Autodesk Fusion 360 part; units mm, degrees
note: some values were not read from the file. Chosen so that the rebuilt part matches the saved one: which bodies a step acts on.
(part 3 of 3)
  line L675 (-34.1437, -40.1697) -> (-31.5928, -38.6629) construction
  line L676 (-31.5928, -38.6629) -> (-29.8835, -37.7222) construction
  spline S219 degree 3 poles (-29.8835, -37.7222) (-29.2848, -37.3926) (-28.7626, -37.0952) (-27.9251, -36.6064) knots 0 0 0 0 1 1 1 1
  line L677 (-29.8835, -37.7222) -> (-29.2848, -37.3926) construction
  line L678 (-29.2848, -37.3926) -> (-28.7626, -37.0952) construction
  line L679 (-28.7626, -37.0952) -> (-27.9251, -36.6064) construction
  spline S220 degree 3 poles (-27.9251, -36.6064) (-26.9048, -36.0111) (-26.2975, -35.6653) (-26.2208, -35.636) knots 0 0 0 0 1 1 1 1
  line L680 (-27.9251, -36.6064) -> (-26.9048, -36.0111) construction
  line L681 (-26.9048, -36.0111) -> (-26.2975, -35.6653) construction
  line L682 (-26.2975, -35.6653) -> (-26.2208, -35.636) construction
  spline S221 degree 3 poles (-26.2208, -35.636) (-26.2038, -35.6296) (-26.0008, -35.7304) (-25.6667, -35.9114) knots 0 0 0 0 1 1 1 1
  line L683 (-26.2208, -35.636) -> (-26.2038, -35.6296) construction
  line L684 (-26.2038, -35.6296) -> (-26.0008, -35.7304) construction
  line L685 (-26.0008, -35.7304) -> (-25.6667, -35.9114) construction
  spline S222 degree 3 poles (-25.7428, -37.5545) (-24.4673, -38.1995) (-21.2005, -40.009) (-19.166, -41.1975) knots 0 0 0 0 1 1 1 1
  line L686 (-25.7428, -37.5545) -> (-24.4673, -38.1995) construction
  line L687 (-24.4673, -38.1995) -> (-21.2005, -40.009) construction
  line L688 (-21.2005, -40.009) -> (-19.166, -41.1975) construction
  spline S223 degree 3 poles (-19.166, -41.1975) (-18.513, -41.5789) (-18.0684, -41.8524) (-18.0809, -41.8648) knots 0 0 0 0 1 1 1 1
  line L689 (-19.166, -41.1975) -> (-18.513, -41.5789) construction
  line L690 (-18.513, -41.5789) -> (-18.0684, -41.8524) construction
  line L691 (-18.0684, -41.8524) -> (-18.0809, -41.8648) construction
  spline S224 degree 3 poles (-18.0809, -41.8648) (-18.1008, -41.8847) (-18.5997, -41.6495) (-19.6279, -41.1354) knots 0 0 0 0 1 1 1 1
  line L692 (-18.0809, -41.8648) -> (-18.1008, -41.8847) construction
  line L693 (-18.1008, -41.8847) -> (-18.5997, -41.6495) construction
  line L694 (-18.5997, -41.6495) -> (-19.6279, -41.1354) construction
  spline S225 degree 3 poles (-19.6279, -41.1354) (-20.9362, -40.4812) (-21.7257, -40.0612) (-22.0995, -39.8204) knots 0 0 0 0 1 1 1 1
  line L695 (-19.6279, -41.1354) -> (-20.9362, -40.4812) construction
  line L696 (-20.9362, -40.4812) -> (-21.7257, -40.0612) construction
  line L697 (-21.7257, -40.0612) -> (-22.0995, -39.8204) construction
  spline S226 degree 3 poles (-22.0995, -39.8204) (-22.4079, -39.6216) (-22.6658, -39.4794) (-23.2646, -39.1777) knots 0 0 0 0 1 1 1 1
  line L698 (-22.0995, -39.8204) -> (-22.4079, -39.6216) construction
  line L699 (-22.4079, -39.6216) -> (-22.6658, -39.4794) construction
  line L700 (-22.6658, -39.4794) -> (-23.2646, -39.1777) construction
  spline S227 degree 3 poles (-23.2646, -39.1777) (-24.0824, -38.7657) (-24.7899, -38.3231) (-25.4378, -38.0628) knots 0 0 0 0 1 1 1 1
  line L701 (-23.2646, -39.1777) -> (-24.0824, -38.7657) construction
  line L702 (-24.0824, -38.7657) -> (-24.7899, -38.3231) construction
  line L703 (-24.7899, -38.3231) -> (-25.4378, -38.0628) construction
  spline S228 degree 3 poles (-25.4378, -38.0628) (-25.9181, -37.8698) (-25.5452, -37.9991) (-26.072, -37.7234) knots 0 0 0 0 1 1 1 1
  line L704 (-25.4378, -38.0628) -> (-25.9181, -37.8698) construction
  line L705 (-25.9181, -37.8698) -> (-25.5452, -37.9991) construction
  line L706 (-25.5452, -37.9991) -> (-26.072, -37.7234) construction
  spline S229 degree 3 poles (-26.072, -37.7234) (-26.2446, -37.6817) (-26.575, -37.8504) (-26.6249, -37.87) knots 0 0 0 0 1 1 1 1
  line L707 (-26.072, -37.7234) -> (-26.2446, -37.6817) construction
  line L708 (-26.2446, -37.6817) -> (-26.575, -37.8504) construction
  line L709 (-26.575, -37.8504) -> (-26.6249, -37.87) construction
  spline S230 degree 3 poles (-26.6249, -37.87) (-26.7469, -37.9178) (-27.123, -38.1964) (-28.1297, -38.7533) knots 0 0 0 0 1 1 1 1
  line L710 (-26.6249, -37.87) -> (-26.7469, -37.9178) construction
  line L711 (-26.7469, -37.9178) -> (-27.123, -38.1964) construction
  line L712 (-27.123, -38.1964) -> (-28.1297, -38.7533) construction
  spline S231 degree 3 poles (-28.1297, -38.7533) (-31.2174, -40.4614) (-33.3065, -41.7393) (-33.8578, -41.9941) knots 0 0 0 0 1 1 1 1
  line L713 (-28.1297, -38.7533) -> (-31.2174, -40.4614) construction
  line L714 (-31.2174, -40.4614) -> (-33.3065, -41.7393) construction
  line L715 (-33.3065, -41.7393) -> (-33.8578, -41.9941) construction
  spline S232 degree 3 poles (-33.8578, -41.9941) (-34.2176, -42.1604) (-34.3437, -42.1895) (-34.3635, -42.1108) knots 0 0 0 0 1 1 1 1
  line L716 (-33.8578, -41.9941) -> (-34.2176, -42.1604) construction
  line L717 (-34.2176, -42.1604) -> (-34.3437, -42.1895) construction
  line L718 (-34.3437, -42.1895) -> (-34.3635, -42.1108) construction
  spline S233 degree 3 poles (-34.3635, -42.1108) (-34.3767, -42.058) (-34.3713, -42.0507) (-34.2413, -41.9471) knots 0 0 0 0 1 1 1 1
  line L719 (-34.3635, -42.1108) -> (-34.3767, -42.058) construction
  line L720 (-34.3767, -42.058) -> (-34.3713, -42.0507) construction
  line L721 (-34.3713, -42.0507) -> (-34.2413, -41.9471) construction
  spline S234 degree 3 poles (-34.2413, -41.9471) (-33.9434, -41.7095) (-33.4673, -41.4178) (-32.2551, -40.7301) knots 0 0 0 0 1 1 1 1
  line L722 (-34.2413, -41.9471) -> (-33.9434, -41.7095) construction
  line L723 (-33.9434, -41.7095) -> (-33.4673, -41.4178) construction
  line L724 (-33.4673, -41.4178) -> (-32.2551, -40.7301) construction
  spline S235 degree 3 poles (-32.2551, -40.7301) (-31.7688, -40.4542) (-30.8392, -39.9239) (-30.1893, -39.5516) knots 0 0 0 0 1 1 1 1
  line L725 (-32.2551, -40.7301) -> (-31.7688, -40.4542) construction
  line L726 (-31.7688, -40.4542) -> (-30.8392, -39.9239) construction
  line L727 (-30.8392, -39.9239) -> (-30.1893, -39.5516) construction
  spline S236 degree 3 poles (-30.1893, -39.5516) (-27.8491, -38.2112) (-27.325, -37.9184) (-26.658, -37.5787) knots 0 0 0 0 1 1 1 1
  line L728 (-30.1893, -39.5516) -> (-27.8491, -38.2112) construction
  line L729 (-27.8491, -38.2112) -> (-27.325, -37.9184) construction
  line L730 (-27.325, -37.9184) -> (-26.658, -37.5787) construction
  spline S237 degree 3 poles (-26.658, -37.5787) (-26.4, -37.4473) (-26.2063, -37.3585) (-26.178, -37.3585) knots 0 0 0 0 1 1 1 1
  line L731 (-26.658, -37.5787) -> (-26.4, -37.4473) construction
  line L732 (-26.4, -37.4473) -> (-26.2063, -37.3585) construction
  line L733 (-26.2063, -37.3585) -> (-26.178, -37.3585) construction
  spline S238 degree 3 poles (-26.178, -37.3585) (-26.15, -37.3585) (-25.9704, -37.4394) (-25.7428, -37.5545) knots 0 0 0 0 1 1 1 1
  line L734 (-26.178, -37.3585) -> (-26.15, -37.3585) construction
  line L735 (-26.15, -37.3585) -> (-25.9704, -37.4394) construction
  line L736 (-25.9704, -37.4394) -> (-25.7428, -37.5545) construction
  spline S239 degree 3 poles (-26.1154, -34.9158) (-25.8921, -34.9929) (-25.0226, -35.4205) (-24.4215, -35.7486) knots 0 0 0 0 1 1 1 1
  line L737 (-26.1154, -34.9158) -> (-25.8921, -34.9929) construction
  line L738 (-25.8921, -34.9929) -> (-25.0226, -35.4205) construction
  line L739 (-25.0226, -35.4205) -> (-24.4215, -35.7486) construction
  spline S240 degree 3 poles (-24.4215, -35.7486) (-24.1169, -35.9149) (-19.3681, -38.5832) (-18.571, -39.0359) knots 0 0 0 0 1 1 1 1
  line L740 (-24.4215, -35.7486) -> (-24.1169, -35.9149) construction
  line L741 (-24.1169, -35.9149) -> (-19.3681, -38.5832) construction
  line L742 (-19.3681, -38.5832) -> (-18.571, -39.0359) construction
  spline S241 degree 3 poles (-18.571, -39.0359) (-17.405, -39.6982) (-16.5172, -40.2351) (-16.5439, -40.2618) knots 0 0 0 0 1 1 1 1
  line L743 (-18.571, -39.0359) -> (-17.405, -39.6982) construction
  line L744 (-17.405, -39.6982) -> (-16.5172, -40.2351) construction
  line L745 (-16.5172, -40.2351) -> (-16.5439, -40.2618) construction
  spline S242 degree 3 poles (-16.5439, -40.2618) (-16.5585, -40.2764) (-16.8618, -40.1363) (-17.3563, -39.8865) knots 0 0 0 0 1 1 1 1
  line L746 (-16.5439, -40.2618) -> (-16.5585, -40.2764) construction
  line L747 (-16.5585, -40.2764) -> (-16.8618, -40.1363) construction
  line L748 (-16.8618, -40.1363) -> (-17.3563, -39.8865) construction
  spline S243 degree 3 poles (-17.3563, -39.8865) (-18.1679, -39.4765) (-19.8684, -38.5676) (-24.1622, -36.2488) knots 0 0 0 0 1 1 1 1
  line L749 (-17.3563, -39.8865) -> (-18.1679, -39.4765) construction
  line L750 (-18.1679, -39.4765) -> (-19.8684, -38.5676) construction
  line L751 (-19.8684, -38.5676) -> (-24.1622, -36.2488) construction
  line L752 (-24.1622, -36.2488) -> (-25.9936, -35.2597)
  line L753 (-25.9936, -35.2597) -> (-26.7073, -35.6419)
  spline S244 degree 3 poles (-26.7073, -35.6419) (-27.8903, -36.2753) (-29.1019, -36.9382) (-31.7923, -38.4243) knots 0 0 0 0 1 1 1 1
  line L754 (-26.7073, -35.6419) -> (-27.8903, -36.2753) construction
  line L755 (-27.8903, -36.2753) -> (-29.1019, -36.9382) construction
  line L756 (-29.1019, -36.9382) -> (-31.7923, -38.4243) construction
  spline S245 degree 3 poles (-31.7923, -38.4243) (-33.9077, -39.5928) (-34.4259, -39.8735) (-34.9611, -40.1412) knots 0 0 0 0 1 1 1 1
  line L757 (-31.7923, -38.4243) -> (-33.9077, -39.5928) construction
  line L758 (-33.9077, -39.5928) -> (-34.4259, -39.8735) construction
  line L759 (-34.4259, -39.8735) -> (-34.9611, -40.1412) construction
  spline S246 degree 3 poles (-34.9611, -40.1412) (-35.4286, -40.375) (-35.6579, -40.4604) (-35.7384, -40.4306) knots 0 0 0 0 1 1 1 1
  line L760 (-34.9611, -40.1412) -> (-35.4286, -40.375) construction
  line L761 (-35.4286, -40.375) -> (-35.6579, -40.4604) construction
  line L762 (-35.6579, -40.4604) -> (-35.7384, -40.4306) construction
  spline S247 degree 3 poles (-35.7384, -40.4306) (-35.8101, -40.4041) (-35.7817, -40.3579) (-35.6306, -40.2549) knots 0 0 0 0 1 1 1 1
  line L763 (-35.7384, -40.4306) -> (-35.8101, -40.4041) construction
  line L764 (-35.8101, -40.4041) -> (-35.7817, -40.3579) construction
  line L765 (-35.7817, -40.3579) -> (-35.6306, -40.2549) construction
  spline S248 degree 3 poles (-35.6306, -40.2549) (-34.7769, -39.6734) (-28.9995, -36.3439) (-26.879, -35.2113) knots 0 0 0 0 1 1 1 1
  line L766 (-35.6306, -40.2549) -> (-34.7769, -39.6734) construction
  line L767 (-34.7769, -39.6734) -> (-28.9995, -36.3439) construction
  line L768 (-28.9995, -36.3439) -> (-26.879, -35.2113) construction
  spline S249 degree 3 poles (-26.879, -35.2113) (-26.2698, -34.8859) (-26.2377, -34.8735) (-26.1154, -34.9158) knots 0 0 0 0 1 1 1 1
  line L769 (-26.879, -35.2113) -> (-26.2698, -34.8859) construction
  line L770 (-26.2698, -34.8859) -> (-26.2377, -34.8735) construction
  line L771 (-26.2377, -34.8735) -> (-26.1154, -34.9158) construction
  spline S250 degree 3 poles (-25.9832, -34.1748) (-25.3061, -34.5036) (-23.6316, -35.4014) (-22.711, -35.9292) knots 0 0 0 0 1 1 1 1
  line L772 (-25.9832, -34.1748) -> (-25.3061, -34.5036) construction
  line L773 (-25.3061, -34.5036) -> (-23.6316, -35.4014) construction
  line L774 (-23.6316, -35.4014) -> (-22.711, -35.9292) construction
  spline S251 degree 3 poles (-22.711, -35.9292) (-22.1528, -36.2492) (-21.7622, -36.4638) (-20.8765, -36.9368) knots 0 0 0 0 1 1 1 1
  line L775 (-22.711, -35.9292) -> (-22.1528, -36.2492) construction
  line L776 (-22.1528, -36.2492) -> (-21.7622, -36.4638) construction
  line L777 (-21.7622, -36.4638) -> (-20.8765, -36.9368) construction
  spline S252 degree 3 poles (-20.8765, -36.9368) (-18.5007, -38.2058) (-16.0738, -39.5933) (-16.1307, -39.6502) knots 0 0 0 0 1 1 1 1
  line L778 (-20.8765, -36.9368) -> (-18.5007, -38.2058) construction
  line L779 (-18.5007, -38.2058) -> (-16.0738, -39.5933) construction
  line L780 (-16.0738, -39.5933) -> (-16.1307, -39.6502) construction
  spline S253 degree 3 poles (-16.1307, -39.6502) (-16.1794, -39.699) (-17.4464, -39.0334) (-21.7111, -36.7188) knots 0 0 0 0 1 1 1 1
  line L781 (-16.1307, -39.6502) -> (-16.1794, -39.699) construction
  line L782 (-16.1794, -39.699) -> (-17.4464, -39.0334) construction
  line L783 (-17.4464, -39.0334) -> (-21.7111, -36.7188) construction
  spline S254 degree 3 poles (-21.7111, -36.7188) (-23.0163, -36.0104) (-23.7493, -35.6248) (-25.0769, -34.9479) knots 0 0 0 0 1 1 1 1
  line L784 (-21.7111, -36.7188) -> (-23.0163, -36.0104) construction
  line L785 (-23.0163, -36.0104) -> (-23.7493, -35.6248) construction
  line L786 (-23.7493, -35.6248) -> (-25.0769, -34.9479) construction
  spline S255 degree 3 poles (-25.0769, -34.9479) (-25.5965, -34.6831) (-26.0305, -34.4663) (-26.0413, -34.4663) knots 0 0 0 0 1 1 1 1
  line L787 (-25.0769, -34.9479) -> (-25.5965, -34.6831) construction
  line L788 (-25.5965, -34.6831) -> (-26.0305, -34.4663) construction
  line L789 (-26.0305, -34.4663) -> (-26.0413, -34.4663) construction
  spline S256 degree 3 poles (-26.0413, -34.4663) (-26.0521, -34.4663) (-26.7797, -34.8596) (-27.6582, -35.3402) knots 0 0 0 0 1 1 1 1
  line L790 (-26.0413, -34.4663) -> (-26.0521, -34.4663) construction
  line L791 (-26.0521, -34.4663) -> (-26.7797, -34.8596) construction
  line L792 (-26.7797, -34.8596) -> (-27.6582, -35.3402) construction
  spline S257 degree 3 poles (-27.6582, -35.3402) (-30.8435, -37.0829) (-31.2781, -37.3146) (-32.1025, -37.7095) knots 0 0 0 0 1 1 1 1
  line L793 (-27.6582, -35.3402) -> (-30.8435, -37.0829) construction
  line L794 (-30.8435, -37.0829) -> (-31.2781, -37.3146) construction
  line L795 (-31.2781, -37.3146) -> (-32.1025, -37.7095) construction
  spline S258 degree 3 poles (-32.1025, -37.7095) (-32.1596, -37.7368) (-32.3046, -37.8236) (-32.4248, -37.9024) knots 0 0 0 0 1 1 1 1
  line L796 (-32.1025, -37.7095) -> (-32.1596, -37.7368) construction
  line L797 (-32.1596, -37.7368) -> (-32.3046, -37.8236) construction
  line L798 (-32.3046, -37.8236) -> (-32.4248, -37.9024) construction
  spline S259 degree 3 poles (-32.4248, -37.9024) (-32.8253, -38.165) (-33.2586, -38.4152) (-34.23, -38.9449) knots 0 0 0 0 1 1 1 1
  line L799 (-32.4248, -37.9024) -> (-32.8253, -38.165) construction
  line L800 (-32.8253, -38.165) -> (-33.2586, -38.4152) construction
  line L801 (-33.2586, -38.4152) -> (-34.23, -38.9449) construction
  spline S260 degree 3 poles (-34.23, -38.9449) (-34.9008, -39.3107) (-35.3686, -39.5733) (-35.6981, -39.769) knots 0 0 0 0 1 1 1 1
  line L802 (-34.23, -38.9449) -> (-34.9008, -39.3107) construction
  line L803 (-34.9008, -39.3107) -> (-35.3686, -39.5733) construction
  line L804 (-35.3686, -39.5733) -> (-35.6981, -39.769) construction
  spline S261 degree 3 poles (-35.6981, -39.769) (-35.9605, -39.9249) (-36.109, -39.9572) (-36.1564, -39.8685) knots 0 0 0 0 1 1 1 1
  line L805 (-35.6981, -39.769) -> (-35.9605, -39.9249) construction
  line L806 (-35.9605, -39.9249) -> (-36.109, -39.9572) construction
  line L807 (-36.109, -39.9572) -> (-36.1564, -39.8685) construction
  spline S262 degree 3 poles (-36.1564, -39.8685) (-36.1729, -39.8378) (-36.1639, -39.8232) (-36.0784, -39.7403) knots 0 0 0 0 1 1 1 1
  line L808 (-36.1564, -39.8685) -> (-36.1729, -39.8378) construction
  line L809 (-36.1729, -39.8378) -> (-36.1639, -39.8232) construction
  line L810 (-36.1639, -39.8232) -> (-36.0784, -39.7403) construction
  spline S263 degree 3 poles (-36.0784, -39.7403) (-35.8332, -39.5028) (-35.075, -39.0535) (-31.6684, -37.1272) knots 0 0 0 0 1 1 1 1
  line L811 (-36.0784, -39.7403) -> (-35.8332, -39.5028) construction
  line L812 (-35.8332, -39.5028) -> (-35.075, -39.0535) construction
  line L813 (-35.075, -39.0535) -> (-31.6684, -37.1272) construction
  spline S264 degree 3 poles (-31.6684, -37.1272) (-29.645, -35.9831) (-29.0122, -35.6236) (-27.9003, -34.987) knots 0 0 0 0 1 1 1 1
  line L814 (-31.6684, -37.1272) -> (-29.645, -35.9831) construction
  line L815 (-29.645, -35.9831) -> (-29.0122, -35.6236) construction
  line L816 (-29.0122, -35.6236) -> (-27.9003, -34.987) construction
  spline S265 degree 3 poles (-27.9003, -34.987) (-26.7253, -34.3142) (-26.2796, -34.0695) (-26.2302, -34.0701) knots 0 0 0 0 1 1 1 1
  line L817 (-27.9003, -34.987) -> (-26.7253, -34.3142) construction
  line L818 (-26.7253, -34.3142) -> (-26.2796, -34.0695) construction
  line L819 (-26.2796, -34.0695) -> (-26.2302, -34.0701) construction
  spline S266 degree 3 poles (-26.2302, -34.0701) (-26.2125, -34.0704) (-26.1014, -34.1175) (-25.9832, -34.1748) knots 0 0 0 0 1 1 1 1
  line L820 (-26.2302, -34.0701) -> (-26.2125, -34.0704) construction
  line L821 (-26.2125, -34.0704) -> (-26.1014, -34.1175) construction
  line L822 (-26.1014, -34.1175) -> (-25.9832, -34.1748) construction
  line L823 (-46, -28) -> (-6, -28)
  line L824 (-6, -28) -> (-6, -30)
  line L825 (-46, -30) -> (-46, -28)
  line L826 (-46, -57) -> (-46, -55)
  line L827 (-6, -55) -> (-6, -57)
  line L828 (-6, -57) -> (-46, -57)
  line L829 (-46, -18) -> (-46, -16)
  line L830 (-46, -16) -> (-6, -16)
  line L831 (-6, -16) -> (-6, -18)
  line L832 (-6, -18) -> (-46, -18)
  line L833 (-46, -22) -> (-46, -20)
  line L834 (-46, -20) -> (-6, -20)
  line L835 (-6, -20) -> (-6, -22)
  line L836 (-6, -22) -> (-46, -22)
  line L837 (-46, -59) -> (-6, -59)
  line L838 (-6, -59) -> (-6, -61)
  line L839 (-6, -61) -> (-46, -61)
  line L840 (-46, -61) -> (-46, -59)
  line L841 (-46, -26) -> (-46, -24)
  line L842 (-46, -24) -> (-6, -24)
  line L843 (-6, -24) -> (-6, -26)
  line L844 (-6, -26) -> (-46, -26)
  line L845 (-46, -63) -> (-6, -63)
  line L846 (-6, -63) -> (-6, -65)
  line L847 (-6, -65) -> (-46, -65)
  line L848 (-46, -65) -> (-46, -63)
fillet "Raccordo2" radius 1 1 edges at (0, 35, 24) on bodies 1
fillet "Raccordo2" radius 1 1 edges at (52, 35, 24) on bodies 1
fillet "Raccordo2" radius 1 1 edges at (0, 35, 0) on bodies 1
fillet "Raccordo2" radius 1 1 edges at (52, 35, 0) on bodies 1
chamfer "Smusso1" distance 5 angle 10 1 edges at (26, 9.8, 22.5) measured on face at (18, 3.2667, 22.5) on bodies 1
chamfer "Smusso1" distance 5 angle 10 1 edges at (26, 9.8, 1.5) measured on face at (34, 3.2667, 1.5) on bodies 1
extrude "Estrusione1''" add sketch "Schizzo12" along normal blind 1.5 separate body contours S0 S1 S2 S3 S4 S5 S6 S7 S8 S9 S10 S11 S12 S13 S14 S15 S16 L57 | S17 S18 S19 S20 S21 S22 S23 S24 S25 S26 S27 | S28 S29 S30 S31 S32 S33 L109 L110 S34 S35 S36 S37 S38 S39 | S40 S41 S42 S43 S44 S45 S46 S47 S48 S49 S50 S51 | S52 S53 S54 S55 S56 S57 S58 S59 S60 S61 S62 S63 S64 S65 | S66 S67 S68 S69 L219 L220 S70 S71 S72 S73 S74 S75 | S76 S77 S78 S79 S80 S81 S82 S83 S84 S85 S86 | S87 S88 L278 L279 S89 S90 S91 S92 S93 S94 S95 S96 S97 | S98 S99 S100 S101 L319 L320 S102 S103 S104 S105 S106 S107 S108 | S109 S110 S111 L351 L352 S112 S113 S114 S115 S116 S117 S118 S119 S120 | S121 S122 S123 S124 S125 S126 S127 S128 S129 | S130 S131 S132 S133 S134 S135 S136 S137 S138 S139 | S140 S141 S142 S143 L449 L450 S144 S145 S146 S147 S148 | S149 S150 S151 S152 S153 S154 S155 S156 S157 S158 S159 | S160 S161 S162 S163 S164 S165 S166 S167 | S168 S169 S170 S171 S172 S173 S174 | S175 S176 S177 S178 | S179 S180 S181 S182 S183 S184 S185 S186 S187 S188 S189 S190 S191 S192 L598 | S193 S194 S195 S196 S197 S198 S199 S200 S201 S202 S203 S204 S205 S206 | S207 S208 S209 S210 S211 S212 S213 S214 S215 S216 S217 S218 S219 S220 S221 | S222 S223 S224 S225 S226 S227 S228 S229 S230 S231 S232 S233 S234 S235 S236 S237 S238 | S239 S240 S241 S242 S243 L752 L753 S244 S245 S246 S247 S248 S249 | S250 S251 S252 S253 S254 S255 S256 S257 S258 S259 S260 S261 S262 S263 S264 S265 S266 makes body 8 at (25.9318, 50.5832, 24.6667) makes body 9 at (28.2629, 48.3854, 24.6667) makes body 10 at (27.7751, 44.7717, 24.6667) makes body 11 at (27.951, 41.5705, 24.6667) makes body 12 at (19.8854, 40.7808, 24.6667) makes body 13 at (20.3981, 37.4305, 24.6667) makes body 14 at (33.9207, 41.2115, 24.6667) makes body 15 at (31.4377, 43.1547, 24.6667) makes body 16 at (26.6178, 43.376, 24.6667) makes body 17 at (28.7885, 47.8461, 24.6667) makes body 18 at (27.1529, 50.2145, 24.6667) makes body 19 at (26.2858, 51.3984, 24.6667) makes body 20 at (25.6562, 48.2288, 24.6667) makes body 21 at (29.9249, 46.8858, 24.6667) makes body 22 at (25.1361, 41.9533, 24.6667) makes body 23 at (25.0536, 38.7124, 24.6667) makes body 24 at (27.7095, 35.6634, 24.6667) makes body 25 at (24.808, 36.3798, 24.6667) makes body 26 at (30.1939, 41.669, 24.6667) makes body 27 at (27.7664, 43.114, 24.6667) makes body 28 at (27.3189, 46.6764, 24.6667) makes body 29 at (25.1472, 49.3364, 25.1667) makes body 30 at (26.0319, 52.1935, 24.6667) in component "Componente_Logo"
ref_plane "Piano di lavoro3" through (26, 70, 12) normal (0, 1, 0) x (-1, 0, 0)
sketch "Schizzo13" plane through (26, 70, 12) normal (0, 1, 0) x (1, 0, 0)
  line L0 (26, -12) -> (-26, -12)
  line L1 (-26, -12) -> (-26, 12)
  line L2 (-26, 12) -> (26, 12)
  line L3 (26, 12) -> (26, -12)
  dimension "d99" = 24
  dimension "d100" = 52
  constraint horizontal L0
  constraint perpendicular L0 L1
  constraint perpendicular L1 L2
  constraint perpendicular L0 L3
  measures "d99" distance of L0.start L2.end
  measures "d100" distance of L0.start L0.end
extrude "Estrusione9" add sketch "Schizzo13" along normal blind 2 separate body makes body 31
sketch "Schizzo14" plane through (0, 72, 0) normal (0, 1, 0) x (-1, 0, 0)
  line L0 (-52, 0) -> (0, 0)
  line L1 (0, 0) -> (0, 24)
  line L2 (0, 24) -> (-52, 24)
  line L3 (-52, 24) -> (-52, 0)
  circle A0 centre (-50, 12.7) radius 0.65
  circle A1 centre (-2, 12.7) radius 0.65
  circle A2 centre (-2, 12.7) radius 0.65
  dimension "d122" = 2
  constraint equal A0 A1
  constraint equal A1 A2
  constraint coincident A1.centre A2.centre
  constraint horizontal A0.centre A1.centre
  measures "d122" distance of L3 A0.centre
hole "Foratura2" at (50, 72, 12.7) at (2, 72, 12.7) direction (0, -1, 0) diameter 1.3 depth 2.097 tip angle 180 countersink diameter 1.6 countersink angle 90 bodies 31
sketch "Schizzo15" plane through (0, 70, 0) normal (0, -1, 0) x (1, 0, 0)
  circle A0 centre (50, 12.7) radius 0.65
  circle A1 centre (2, 12.7) radius 0.65
  line L0 (0, 0) -> (52, 0)
  line L1 (52, 0) -> (52, 24)
  line L2 (52, 24) -> (0, 24)
  line L3 (0, 24) -> (0, 0)
  line L4 (5, 9.85) -> (47, 9.85)
  line L5 (47, 9.85) -> (47, 7.85)
  line L6 (47, 7.85) -> (5, 7.85)
  line L7 (5, 7.85) -> (5, 9.85)
  line L8 (5, 9.85) -> (47, 9.85)
  line L9 (5, 7.85) -> (5, 9.85)
  constraint horizontal L4
  constraint vertical L5
  constraint horizontal L6
  constraint vertical L7
  constraint equal L4 L8
  constraint equal L7 L9
  constraint coincident L4.start L7.end
extrude "Estrusione10" add sketch "Schizzo15" along normal blind 1.4 contours L4 L5 L6 L7 L8 L9 bodies 31
fillet "Raccordo3" radius 1 1 edges at (52, 71, 24) on bodies 31
fillet "Raccordo3" radius 1 1 edges at (0, 71, 24) on bodies 31
fillet "Raccordo3" radius 1 1 edges at (52, 71, 0) on bodies 31
fillet "Raccordo3" radius 1 1 edges at (0, 71, 0) on bodies 31
copy_body "Corpo->Comp1" bodies 31 removing the originals makes body 32 in component "Coperchio"
copy_body "Corpo->Comp2" bodies 1 removing the originals makes body 33 in component "Case"
other "Lavorazione mesh di base1"
other "Corpo->Comp1'"
other "Modifica1" in component "pcb-MultiRom"
other "Lavorazione mesh di base2"
other "Corpo->Comp2'"
other "Modifica1'" in component "edgeconnector-Model"
other "Modifica2" in component "edgeconnector-Model"
combine "Combina2" operation add target body 33 tool bodies 4 7 5 6 2 3 in component "Case"
sketch "Schizzo16" plane through (0, 0, 24) normal (0, 0, 1) x (-1, 0, 0)
  line L0 (-16.0196, -48.0156) -> (-16.0196, -48.6944)
  line L1 (-17.5571, -48.6944) -> (-17.5571, -46.2033)
  spline S0 degree 2 poles (-17.5571, -46.2033) (-16.8532, -45.9324) (-16.0939, -45.9324) knots 0 0 0 1 1 1
  spline S1 degree 2 poles (-16.0939, -45.9324) (-15.19, -45.9324) (-14.6849, -46.6156) knots 0 0 0 1 1 1
  spline S2 degree 2 poles (-14.6849, -46.6156) (-14.1799, -47.2988) (-14.1799, -48.4965) knots 0 0 0 1 1 1
  spline S3 degree 2 poles (-14.1799, -48.4965) (-14.1799, -49.6843) (-14.7346, -50.3675) knots 0 0 0 1 1 1
  spline S4 degree 2 poles (-14.7346, -50.3675) (-15.2893, -51.0507) (-16.2629, -51.0507) knots 0 0 0 1 1 1
  spline S5 degree 2 poles (-16.2629, -51.0507) (-16.9168, -51.0507) (-17.4809, -50.7257) knots 0 0 0 1 1 1
  line L2 (-17.4809, -50.7257) -> (-17.2047, -50.0935)
  spline S6 degree 2 poles (-17.2047, -50.0935) (-16.669, -50.3719) (-16.2445, -50.3719) knots 0 0 0 1 1 1
  spline S7 degree 2 poles (-16.2445, -50.3719) (-15.647, -50.3719) (-15.3092, -49.8807) knots 0 0 0 1 1 1
  spline S8 degree 2 poles (-15.3092, -49.8807) (-14.9715, -49.3894) (-14.9715, -48.4915) knots 0 0 0 1 1 1
  spline S9 degree 2 poles (-14.9715, -48.4915) (-14.9715, -46.6112) (-16.2022, -46.6112) knots 0 0 0 1 1 1
  spline S10 degree 2 poles (-16.2022, -46.6112) (-16.5151, -46.6112) (-16.802, -46.6906) knots 0 0 0 1 1 1
  line L3 (-16.802, -46.6906) -> (-16.802, -48.0156)
  line L4 (-16.802, -48.0156) -> (-16.0196, -48.0156)
  line L5 (-13.1262, -46.5373) -> (-13.1262, -46)
  line L6 (-13.1262, -46) -> (-10.4187, -46)
  line L7 (-10.4187, -46) -> (-10.4187, -46.5376)
  line L8 (-10.4187, -46.5376) -> (-11.3966, -46.6039)
  line L9 (-11.3966, -46.6039) -> (-11.3966, -50.3747)
  line L10 (-11.3966, -50.3747) -> (-10.4187, -50.441)
  line L11 (-10.4187, -50.441) -> (-10.4187, -50.9797)
  line L12 (-10.4187, -50.9797) -> (-13.1262, -50.9797)
  line L13 (-13.1262, -50.9797) -> (-13.1262, -50.4413)
  line L14 (-13.1262, -50.4413) -> (-12.1517, -50.3751)
  line L15 (-12.1517, -50.3751) -> (-12.1517, -46.6036)
  line L16 (-12.1517, -46.6036) -> (-13.1262, -46.5373)
  line L17 (-35.9453, -47.9983) -> (-35.2961, -47.9983)
  line L18 (-35.2961, -47.9983) -> (-35.2961, -46)
  line L19 (-35.2961, -46) -> (-34.5409, -46)
  line L20 (-34.5409, -46) -> (-34.5409, -50.9797)
  line L21 (-34.5409, -50.9797) -> (-35.792, -50.9797)
  spline S11 degree 2 poles (-35.792, -50.9797) (-37.5869, -50.9797) (-37.5869, -49.5355) knots 0 0 0 1 1 1
  spline S12 degree 2 poles (-37.5869, -49.5355) (-37.5869, -48.5363) (-36.6274, -48.1996) knots 0 0 0 1 1 1
  line L22 (-36.6274, -48.1996) -> (-37.9461, -46)
  line L23 (-37.9461, -46) -> (-37.1091, -46)
  line L24 (-37.1091, -46) -> (-35.9453, -47.9983)
  spline S13 degree 2 poles (-45.3576, -49.0077) (-45.3576, -49.2263) (-45.3766, -49.6687) knots 0 0 0 0.640385 0.640385 0.640385
  line L25 (-45.3766, -49.6687) -> (-44.5647, -46)
  line L26 (-44.5647, -46) -> (-43.9423, -46)
  line L27 (-43.9423, -46) -> (-43.1615, -49.596)
  spline S14 degree 2 poles (-43.1615, -49.596) (-43.1806, -49.2202) (-43.1806, -48.9646) knots 0.433911 0.433911 0.433911 1 1 1
  line L28 (-43.1806, -48.9646) -> (-43.1806, -46)
  line L29 (-43.1806, -46) -> (-42.5382, -46)
  line L30 (-42.5382, -46) -> (-42.5382, -50.9797)
  line L31 (-42.5382, -50.9797) -> (-43.4818, -50.9797)
  line L32 (-43.4818, -50.9797) -> (-44.2572, -47.2526)
  line L33 (-44.2572, -47.2526) -> (-45.0388, -50.9797)
  line L34 (-45.0388, -50.9797) -> (-46, -50.9797)
  line L35 (-46, -50.9797) -> (-46, -46)
  line L36 (-46, -46) -> (-45.3576, -46)
  line L37 (-45.3576, -46) -> (-45.3576, -49.0077)
  line L38 (-6, -30) -> (-46, -30)
  line L39 (-46, -55) -> (-6, -55)
  line L40 (-51, 0) -> (-51, -70)
  line L41 (-51, -70) -> (-1, -70)
  line L42 (-1, -70) -> (-1, 0)
  line L43 (-1, 0) -> (-51, 0)
  spline S15 degree 2 poles (-8.5566, -48.6203) (-9.4618, -48.3879) (-9.4618, -47.4715) knots 0.093077 0.093077 0.093077 1 1 1
  spline S16 degree 2 poles (-9.4618, -47.4715) (-9.4618, -46.7868) (-9.0172, -46.3934) knots 0 0 0 1 1 1
  spline S17 degree 2 poles (-9.0172, -46.3934) (-8.5725, -46) (-7.8154, -46) knots 0 0 0 1 1 1
  line L44 (-7.8154, -46) -> (-6, -46)
  line L45 (-6, -46) -> (-6, -50.9797)
  line L46 (-6, -50.9797) -> (-7.5273, -50.9797)
  spline S18 degree 2 poles (-7.5273, -50.9797) (-8.4582, -50.9797) (-8.8924, -50.6722) knots 0 0 0 1 1 1
  spline S19 degree 2 poles (-8.8924, -50.6722) (-9.3266, -50.3647) (-9.3266, -49.685) knots 0 0 0 1 1 1
  spline S20 degree 2 poles (-9.3266, -49.685) (-9.3266, -49.2344) (-9.0486, -48.9336) knots 0 0 0 1 1 1
  spline S21 degree 2 poles (-9.0486, -48.9336) (-8.8398, -48.7075) (-8.5566, -48.6203) knots 0 0 0 0.751565 0.751565 0.751565
  spline S22 degree 2 poles (-41.5117, -46.606) (-41.0372, -45.9324) (-40.1538, -45.9324) knots 0 0 0 1 1 1
  spline S23 degree 2 poles (-40.1538, -45.9324) (-38.3215, -45.9324) (-38.3215, -48.5032) knots 0 0 0 1 1 1
  spline S24 degree 2 poles (-38.3215, -48.5032) (-38.3215, -51.0575) (-40.1604, -51.0575) knots 0 0 0 1 1 1
  spline S25 degree 2 poles (-40.1604, -51.0575) (-41.0466, -51.0575) (-41.5164, -50.385) knots 0 0 0 1 1 1
  spline S26 degree 2 poles (-41.5164, -50.385) (-41.9861, -49.7124) (-41.9861, -48.4966) knots 0 0 0 1 1 1
  spline S27 degree 2 poles (-41.9861, -48.4966) (-41.9861, -47.2795) (-41.5117, -46.606) knots 0 0 0 1 1 1
  line L47 (-17.5571, -55) -> (-17.5571, -30) construction
  line L48 (-34.5409, -55) -> (-34.5409, -30) construction
  line L49 (-26, -52.5) -> (-14.5333, -38.625)
  line L50 (-26, -55) -> (-26, -30) construction
  line L51 (-14.5333, -38.625) -> (-26, -32.5)
  line L52 (-26, -52.5) -> (-37.4667, -38.625)
  line L53 (-37.4667, -38.625) -> (-26, -32.5)
  line L54 (-17.5571, -55) -> (-34.5409, -55) construction
  line L55 (-34.5409, -55) -> (-34.5409, -52.5) construction
  line L56 (-34.5409, -52.5) -> (-17.5571, -52.5) construction
  line L57 (-17.5571, -52.5) -> (-17.5571, -55) construction
  line L58 (-17.5571, -30) -> (-34.5409, -30) construction
  line L59 (-34.5409, -30) -> (-34.5409, -32.5) construction
  line L60 (-34.5409, -32.5) -> (-17.5571, -32.5) construction
  line L61 (-17.5571, -32.5) -> (-17.5571, -30) construction
  line L62 (-46, -28) -> (-6, -28)
  line L63 (-6, -28) -> (-6, -30)
  line L64 (-46, -30) -> (-46, -28)
  line L65 (-46, -57) -> (-46, -55)
  line L66 (-6, -55) -> (-6, -57)
  line L67 (-6, -57) -> (-46, -57)
  line L68 (-46, -18) -> (-46, -16)
  line L69 (-46, -16) -> (-6, -16)
  line L70 (-6, -16) -> (-6, -18)
  line L71 (-6, -18) -> (-46, -18)
  line L72 (-46, -22) -> (-46, -20)
  line L73 (-46, -20) -> (-6, -20)
  line L74 (-6, -20) -> (-6, -22)
  line L75 (-6, -22) -> (-46, -22)
  line L76 (-46, -59) -> (-6, -59)
  line L77 (-6, -59) -> (-6, -61)
  line L78 (-6, -61) -> (-46, -61)
  line L79 (-46, -61) -> (-46, -59)
  line L80 (-46, -26) -> (-46, -24)
  line L81 (-46, -24) -> (-6, -24)
  line L82 (-6, -24) -> (-6, -26)
  line L83 (-6, -26) -> (-46, -26)
  line L84 (-46, -63) -> (-6, -63)
  line L85 (-6, -63) -> (-6, -65)
  line L86 (-6, -65) -> (-46, -65)
  line L87 (-46, -65) -> (-46, -63)
  dimension "d129" = 18
  dimension "d139" = 18
  dimension "d140" = 13
  dimension "d141" = 13
  dimension "d142" = 2.5
  constraint coincident L39 L47.start
  constraint perpendicular L39 L47
  constraint coincident L39 L48.start
  constraint coincident L38 L48.end
  constraint perpendicular L38 L48
  constraint midpoint L39 L50.start
  constraint midpoint L38 L50.end
  constraint coincident L50 L51.end
  constraint coincident L49.start L50
  constraint collinear L1 L47
  constraint collinear L20 L48
  constraint horizontal L54
  constraint vertical L55
  constraint horizontal L56
  constraint vertical L57
  constraint coincident L48 L55.end
  constraint horizontal L58
  constraint vertical L59
  constraint horizontal L60
  constraint vertical L61
  constraint coincident L48 L59.end
  constraint coincident L51.end L60
  constraint coincident L49.start L56
  constraint equal L55 L59
  constraint collinear L38 L58
  measures "d129" distance of L49.start L52.end
  measures "d139" distance of L49.start L49.end
  measures "d140" distance of L51.end L49.end
  measures "d141" distance of L51.end L52.end
  measures "d142" distance of L47.end L60.end
extrude "Estrusione1'''" add sketch "Schizzo16" along normal blind 1.5 contours L49 L51 L52 L53 bodies 33 in component "Case"
sketch "Schizzo17" plane through (0, 0, 25.5) normal (0, 0, 1) x (-1, 0, 0)
  line L0 (-26, -52.5) -> (-14.5333, -38.625)
  line L1 (-14.5333, -38.625) -> (-26, -32.5)
  line L2 (-26, -32.5) -> (-37.4667, -38.625)
  line L3 (-37.4667, -38.625) -> (-26, -52.5)
  line L4 (-26, -52.5) -> (-26, -32.5) construction
  line L5 (-22.1778, -47.875) -> (-26, -45.8333)
  line L6 (-26, -45.8333) -> (-29.8222, -47.875)
  line L7 (-23.4519, -49.4167) -> (-26, -48.0556)
  line L8 (-26, -48.0556) -> (-28.5481, -49.4167)
  line L9 (-24.7259, -50.9583) -> (-26, -50.2778)
  line L10 (-26, -50.2778) -> (-27.2741, -50.9583)
  line L11 (-20.9037, -46.3333) -> (-26, -43.6111)
  line L12 (-31.0963, -46.3333) -> (-26, -43.6111)
  line L13 (-19.6296, -44.7917) -> (-26, -41.3889)
  line L14 (-26, -41.3889) -> (-32.3704, -44.7917)
  line L15 (-18.3556, -43.25) -> (-26, -39.1667)
  line L16 (-26, -39.1667) -> (-33.6444, -43.25)
  line L17 (-17.0815, -41.7083) -> (-26, -36.9444)
  line L18 (-26, -36.9444) -> (-34.9185, -41.7083)
  line L19 (-15.8074, -40.1667) -> (-26, -34.7222)
  line L20 (-26, -34.7222) -> (-36.1926, -40.1667)
  line L21 (-15.8074, -40.1667) -> (-17.0815, -41.7083)
  line L22 (-18.3556, -43.25) -> (-19.6296, -44.7917)
  line L23 (-20.9037, -46.3333) -> (-22.1778, -47.875)
  line L24 (-23.4519, -49.4167) -> (-24.7259, -50.9583)
  line L25 (-27.2741, -50.9583) -> (-28.5481, -49.4167)
  line L26 (-29.8222, -47.875) -> (-31.0963, -46.3333)
  line L27 (-32.3704, -44.7917) -> (-33.6444, -43.25)
  line L28 (-34.9185, -41.7083) -> (-36.1926, -40.1667)
  dimension "d132" = 2
  dimension "d133" = 2
  dimension "d134" = 2
  dimension "d135" = 2
  dimension "d136" = 2
  dimension "d137" = 2
  dimension "d138" = 2
  dimension "d143" = 2
  constraint coincident L0.start L3.end
  constraint coincident L1.end L2.start
  constraint coincident L0 L5.start
  constraint coincident L4 L5.end
  constraint coincident L3 L6.end
  constraint coincident L4 L7.end
  constraint coincident L0 L9.start
  constraint coincident L3 L10.end
  constraint parallel L1 L5
  constraint parallel L2 L6
  constraint parallel L5 L7
  constraint parallel L7 L9
  constraint coincident L4 L9.end
  constraint coincident L0 L7.start
  constraint equal L7 L8
  constraint coincident L0 L11.start
  constraint coincident L4 L11.end
  constraint coincident L3 L12.start
  constraint coincident L0 L13.start
  constraint coincident L4 L13.end
  constraint parallel L11 L13
  constraint coincident L3 L14.end
  constraint parallel L12 L14
  constraint parallel L5 L11
  constraint parallel L6 L12
  constraint coincident L0 L15.start
  constraint coincident L4 L15.end
  constraint parallel L13 L15
  constraint coincident L3 L16.end
  constraint coincident L0 L17.start
  constraint coincident L4 L17.end
  constraint parallel L15 L17
  constraint coincident L3 L18.end
  constraint parallel L14 L16
  constraint parallel L16 L18
  constraint coincident L0 L19.start
  constraint coincident L4 L19.end
  constraint coincident L3 L20.end
  constraint parallel L17 L19
  constraint parallel L18 L20
  constraint parallel L3 L25
  constraint equal L9 L10
  measures "d132" distance of L0.start L9.start
  measures "d133" distance of L5.start L7.start
  measures "d134" distance of L7.start L9.start
  measures "d135" distance of L11.start L13.start
  measures "d136" distance of L5.start L11.start
  measures "d137" distance of L13.start L15.start
  measures "d138" distance of L15.start L17.start
  measures "d143" distance of L0.end L19.start
extrude "Estrusione2'" cut sketch "Schizzo17" against normal blind 1.5 contours L0 L3 L7 L8 L9 L10 L24 L25 | L0 L3 L5 L6 L11 L12 L23 L26 | L0 L3 L13 L14 L15 L16 L22 L27 | L0 L3 L17 L18 L19 L20 L21 L28 bodies 33 in component "Case"
component "Componente_Testo" placed x (1, 0, 0) y (0, 1, 0) z (0, 0, 1) at (0, 0, 0)
component "Componente_Logo" placed x (1, 0, 0) y (0, 1, 0) z (0, 0, 1) at (0, 0, 0)
component "Coperchio" placed x (1, 0, 0) y (0, 1, 0) z (0, 0, 1) at (0, 0, 0)
component "Case" placed x (1, 0, 0) y (0, 1, 0) z (0, 0, 1) at (0, 0, 0)
component "pcb-MultiRom" placed x (1, 0, 0) y (0, 1, 0) z (0, 0, 1) at (0, -0.7, 0)
component "edgeconnector-Model" placed x (1, 0, 0) y (0, 1, 0) z (0, 0, 1) at (-4.5, 9.5, 0)
named bodies: "Case", "Coperchio"
